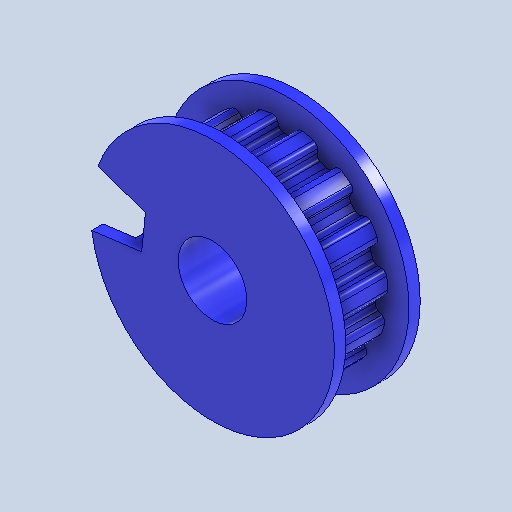
# Autodesk Inventor part: 歯付きプーリ1
Saved by Autodesk Inventor 2025.2 (Build 292293000, 293)
## iProperties
CustomPartVersion: 1
Created: 2025-01-13
Part Number: 歯付きプーリ1
Material: ABS プラスチック
Document SubType Name: Modeling
Designer: haruy
Density: 1.06 g/cm^3
Appearance: 青 - 壁塗料 - 光沢
Author: haruy
Autodesk Inventor part; units mm, degrees
ref_plane "YZ Plane" through (0, 0, 0) normal (1, 0, 0) x (0, 1, 0)
ref_plane "XZ Plane" through (0, 0, 0) normal (0, 1, 0) x (-1, 0, 0)
ref_plane "XY Plane" through (0, 0, 0) normal (0, 0, 1) x (1, 0, 0)
sketch "プーリ スケッチ" plane through (0, 0, 0) normal (0, 0, 1) x (1, 0, 0)
  circle A0 centre (0, 0) radius 22.7393 construction
  circle A1 centre (0, 0) radius 22.3583
  circle A2 centre (0, 0) radius 19.6913
  line L0 (-2.4459, 22.2241) -> (-1.524, 19.6913)
  line L1 (-1.524, 19.6913) -> (1.524, 19.6913)
  line L2 (1.524, 19.6913) -> (2.4459, 22.2241)
  line L3 (0, 0) -> (0, 22.3583) construction
  point P0 (0, 19.6913)
  dimension "d0" = 45.4785
  dimension "d1" = 0.381
  dimension "d2" = 2.667
  dimension "d3" = 40
  dimension "d4" = 3.048
  constraints: 8 end point, 3 coincident, 3 point on circle, 2 centre point, 1 horizontal, 1 midpoint, 1 point on line, 1 vertical, 1 vertical alignment, 3 other
  measures "d0" diameter of A0
  measures "d1" radial gap between concentric circles of A0 A1
  measures "d3" angle of L2 L0
  measures "d4" distance of L0.end L1.end
extrude "基本ボディ" add sketch "プーリ スケッチ" along normal mid plane 14 contours A2 | A1 L0 L1 L2 | L2 L1 L0 A1
extrude "歯" cut sketch "プーリ スケッチ" along normal through all both and the other way through all contours L2 L1 L0 A1 picked at (0, 21.4594)
fillet "Fillet" radius 1.1938 2 edges at (1.524, 19.6913, 0) (-1.524, 19.6913, 0)
fillet "Fillet" radius 1.1684 4 edges at (-2.4459, 22.2241, 3.5) (-2.4459, 22.2241, -3.5) (2.4459, 22.2241, 3.5) (2.4459, 22.2241, -3.5)
pattern_circular "Teeth" count 15 over 360 about axis through (0, 0, -10) along (0, 0, 1) of "歯", "Fillet"
sketch "スケッチ3" plane through (0, 0, -7) normal (0, 0, -1) x (-1, 0, 0)
  circle A0 centre (0, 0) radius 27
  dimension "d18" = 54
  constraints: 1 centre point, 1 coincident
  measures "d18" diameter of A0
extrude "押し出し3" add sketch "スケッチ3" along normal blind 2.5
sketch "スケッチ4" plane through (0, 0, 7) normal (0, 0, 1) x (1, 0, 0)
  circle A0 centre (0, 0) radius 7.6
  circle A1 centre (0, 0) radius 14.5
  circle A2 centre (0, -14.5) radius 1.6
  circle A3 centre (0, 14.5) radius 1.6
  dimension "d22" = 29
  dimension "d21" = 15.2
  dimension "d23" = 3.2
  dimension "d26" = 360
  constraints: 3 centre point, 2 coincident, 1 vertical alignment, 7 other
  measures "d21" diameter of A0
  measures "d23" diameter of A2
extrude "押し出し4" cut sketch "スケッチ4" against normal through all contours A0
sketch "スケッチ5" plane through (0, 0, 7) normal (0, 0, 1) x (1, 0, 0)
  arc A0 (-22.0675, 3.5943) -> (-22.3325, 1.0723) centre (0, 0) ccw projected
  circle A1 centre (0, 0) radius 22.3583
  line L0 (-22.3325, 1.0723) -> (-22.0675, 3.5943)
  line L1 (-22.4327, 0.4636) -> (-21.9228, 5.3144)
  line L2 (-22.6539, -1.641) -> (-21.8177, 6.3152)
  line L3 (-21.8177, 6.3152) -> (-14.856, 5.5835)
  line L4 (-14.856, 5.5835) -> (-15.6922, -2.3727)
  line L5 (-15.6922, -2.3727) -> (-22.6539, -1.641)
  circle A2 centre (0, 0) radius 27.4737
  line L6 (-14.856, 5.5835) -> (-25.8121, 9.4095)
  line L7 (-22.2, 2.3333) -> (0, 0)
  line L8 (-15.6922, -2.3727) -> (-27.2044, -3.8372)
  point P0 (-27.2044, -3.8372)
  dimension "d30" = 7
  dimension "d31" = 8
  dimension "d32" = 4
  dimension "d33" = 13.25
  constraints: 18 end point, 3 parallel, 2 coincident, 2 perpendicular, 2 point on line, 1 midpoint, 1 symmetric about line, 1 tangent, 6 other
  measures "d30" distance of L2.end L3.end
  measures "d31" distance between parallel lines of L3 L5
  measures "d32" distance from line of L5 L7.start
extrude "押し出し5" cut sketch "スケッチ5" against normal through all contours L0 A0 | A0 L1 L2 L3 A1 | A1 L3 L4 L7 L0 | A0 A1 L5 L2 L1 | L1 L2 L5 A1 L8 A2 L6 L3 | A1 L6 L3 | L7 L4 L5 A1 L0 | L5 L8 A1
sketch "スケッチ6" plane through (0, 0, -9.5) normal (0, 0, -1) x (-1, 0, 0)
  line L0 (14.856, 5.5835) -> (25.3649, 9.2533) projected
  arc A0 (25.3649, 9.2533) -> (26.7344, -3.7775) centre (0, 0) ccw projected
  line L1 (26.7344, -3.7775) -> (15.6922, -2.3727) projected
  line L2 (15.6922, -2.3727) -> (14.856, 5.5835) projected
  circle A1 centre (0, 0) radius 7.6 projected
ref_plane "作業平面1" through (0, 0, 0) normal (0, 0, 1) x (1, 0, 0)
mirror "ミラー1" about plane through (0, 0, 0) normal (0, 0, 1) of "押し出し3", "押し出し4", "押し出し5"
equation "\"d1\" = da_a"
equation "\"d2\" = da_hg"
equation "\"d3\" = 2 * da_fi"
equation "\"d4\" = da_bw"
equation "\"d5\" = da_bf"
equation "\"d7\" = da_bf"
equation "\"d9\" = da_rb"
equation "\"d10\" = da_rt"
equation "\"da_pb\" = 9.525"
equation "\"da_fi\" = 20deg"
equation "\"da_hg\" = 2.667"
equation "\"da_bw\" = 3.048"
equation "\"da_rb\" = 1.1938"
equation "\"da_rt\" = 1.1684"
equation "\"da_a\" = 0.381"
equation "\"da_bf\" = 14"
equation "\"da_wf\" = 1.27"
equation "\"da_hf\" = 1.651"
body "Solid1"
